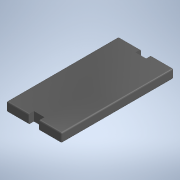
# Autodesk Inventor part: Test2
Saved by Autodesk Inventor 2020 (Build 240168000, 168)
## iProperties
Part Number: Test2
Material: Типовой
Document SubType Name: Обычные детали
Designer: User
Appearance: По умолчанию
Author: User
Autodesk Inventor part; units mm, degrees
ref_plane "Плоскость YZ" through (0, 0, 0) normal (1, 0, 0) x (0, 1, 0)
ref_plane "Плоскость XZ" through (0, 0, 0) normal (0, 1, 0) x (-1, 0, 0)
ref_plane "Плоскость XY" through (0, 0, 0) normal (0, 0, 1) x (1, 0, 0)
sketch "Эскиз1" plane through (0, 0, 0) normal (0, 1, 0) x (-1, 0, 0)
  line L0 (10.9667, 22.3) -> (-10.9667, 22.3)
  line L1 (-10.9667, 22.3) -> (-10.9667, -22.3)
  line L2 (-10.9667, -22.3) -> (10.9667, -22.3)
  line L3 (10.9667, -22.3) -> (10.9667, 22.3)
  line L4 (10.9667, 22.3) -> (-10.9667, -22.3) construction
  line L5 (-10.9667, 22.3) -> (10.9667, -22.3) construction
  point P0 (0, 0)
  dimension "d0" = 44.6
  dimension "d1" = 21.9333
  constraints: 12 end point, 2 midpoint, 2 parallel, 1 horizontal, 1 perpendicular
  measures "d0" distance of L0.end L1.end
  measures "d1" distance between parallel lines of L1 L3
extrude "Выдавливание1" add sketch "Эскиз1" along normal blind 3.58
fillet "Сопряжение1" radius 0.5 12 edges at (0, 3.58, 22.3) (0, 0, 22.3) (10.9667, 1.79, 22.3) (-10.9667, 1.79, 22.3) (-10.9667, 3.58, 0) (10.9667, 3.58, 0) (10.9667, 0, 0) (-10.9667, 0, 0) (0, 3.58, -22.3) (0, 0, -22.3) (-10.9667, 1.79, -22.3) (10.9667, 1.79, -22.3)
sketch "Эскиз2" plane through (0, 3.58, 0) normal (0, 1, 0) x (1, 0, 0)
  line L0 (-2.1, 24.4) -> (2.1, 24.4)
  line L1 (2.1, 24.4) -> (2.1, 20.2)
  line L2 (2.1, 20.2) -> (-2.1, 20.2)
  line L3 (-2.1, 20.2) -> (-2.1, 24.4)
  line L4 (10.4667, 22.3) -> (-10.4667, 22.3) projected
  line L5 (-2.1, 24.4) -> (2.1, 20.2) construction
  line L6 (2.1, 24.4) -> (-2.1, 20.2) construction
  point P0 (0, 0)
  point P1 (0, 22.3)
  dimension "d5" = 4.2
  dimension "d6" = 4.2
  constraints: 12 end point, 3 midpoint, 2 parallel, 1 horizontal, 1 perpendicular
  measures "d5" distance of L0.start L0.end
  measures "d6" distance of L0.end L1.end
extrude "Выдавливание2" cut sketch "Эскиз2" against normal blind 10
mirror "Зеркальное отражение1" about plane through (0, 0, 0) normal (0, 0, 1) of "Выдавливание2"
